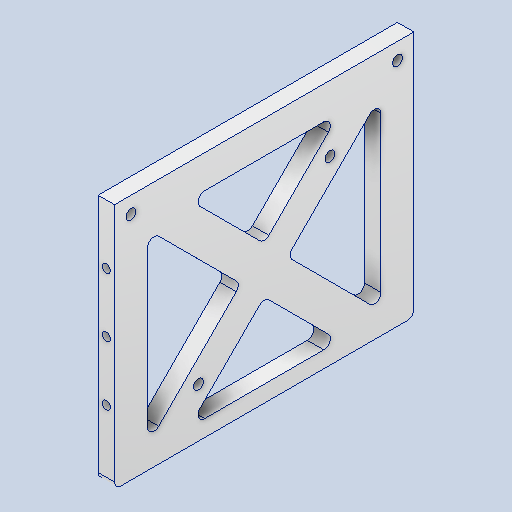
# Autodesk Inventor part: base_weel-v2-Plate-5
Saved by Autodesk Inventor 2025.2 (Build 292293000, 293)
## iProperties
Created: 2025-01-14
Part Number: base_weel-v2-Plate-5
Material: アルミニウム 6061
Document SubType Name: Modeling
Designer: haruy
Density: 2.7 g/cm^3
Appearance: アルミニウム - フラット
Author: haruy
Autodesk Inventor part; units mm, degrees
ref_plane "YZ Plane" through (0, 0, 0) normal (1, 0, 0) x (0, 1, 0)
ref_plane "XZ Plane" through (0, 0, 0) normal (0, 1, 0) x (-1, 0, 0)
ref_plane "XY Plane" through (0, 0, 0) normal (0, 0, 1) x (1, 0, 0)
derived "base_weel-v2-Sketch-Base.ipt"
sketch "スケッチ1" plane through (0, 0, 0) normal (1, 0, 0) x (0, 1, 0)
  line L0 (-315, 315) -> (315, 315)
  line L1 (315, 315) -> (315, -315)
  line L2 (315, -315) -> (-315, -315)
  line L3 (-315, -315) -> (-315, 315)
  line L4 (-315, 315) -> (315, -315) construction
  line L5 (315, 315) -> (-315, -315) construction
  line L6 (-295, 218) -> (-295, -202)
  line L7 (-295, -202) -> (-315, -202)
  line L8 (-315, -202) -> (-315, 210)
  line L9 (242, 315) -> (-242, 315)
  line L10 (-242, 315) -> (-242, 295)
  line L11 (-242, 295) -> (242, 295)
  line L12 (242, 295) -> (242, 315)
  line L13 (-295, 218) -> (-295, 315)
  line L14 (0, 0) -> (-956.5973, 0)
  circle A0 centre (0, 0) radius 400
  line L15 (-330, 25) -> (-380, 25)
  line L16 (-380, 25) -> (-380, -25)
  line L17 (-380, -25) -> (-330, -25)
  line L18 (-330, -25) -> (-330, 25)
  line L19 (0, 0) -> (0, -630.9179)
  line L20 (-315, 40) -> (-395, 40) construction
  line L21 (-395, 40) -> (-395, 30)
  line L22 (-395, 30) -> (-315, 30)
  line L23 (-315, 30) -> (-315, 40)
  line L24 (-395, 30) -> (-385, 30)
  line L25 (-385, 30) -> (-385, 0)
  line L26 (-385, 0) -> (-395, 0)
  line L27 (-395, 0) -> (-395, 30)
  line L28 (295, 202) -> (315, 202)
  line L29 (315, 202) -> (315, -202)
  line L30 (315, -202) -> (295, -202)
  line L31 (295, -202) -> (295, 202)
  line L32 (-222.2183, -315) -> (242, -315)
  line L33 (242, -315) -> (242, -295)
  line L34 (242, -295) -> (-242, -295)
  line L35 (315, 315) -> (0, 0)
  line L36 (315, 125) -> (315, 145)
  circle A1 centre (512, 0) radius 122.5
  circle A2 centre (179.6905, 0) radius 600
  circle A3 centre (541.6815, 0) radius 200
  circle A4 centre (0, 0) radius 10
  arc A5 (0, 150) -> (0, -150) centre (0, 0) ccw
  arc A6 (0, 140) -> (0, -140) centre (0, 0) ccw
  line L37 (-146.3272, 32.9904) -> (-136.572, 30.791)
  line L38 (-137.5812, 37.6817) -> (-140.4404, 25)
  line L39 (-140.4404, 25) -> (-145.318, 26.0997)
  line L40 (-145.318, 26.0997) -> (-142.4588, 38.7814)
  line L41 (-142.4588, 38.7814) -> (-137.5812, 37.6817)
  arc A7 (-29.1302, 142.0438) -> (-29.1302, -142.0438) centre (0, 0) ccw
  circle A8 centre (-151.4904, 39.2799) radius 6.5
  circle A9 centre (-129.0401, 34.2184) radius 6.5 construction
  circle A10 centre (-129.0401, 34.2184) radius 1.5 construction
  circle A11 centre (-151.4904, 39.2799) radius 1.5
  line L42 (-30.1668, 22.5) -> (-174.1362, 22.5)
  line L43 (-174.1362, 22.5) -> (-174.1362, 7.5)
  line L44 (-174.1362, 7.5) -> (-30.1668, 7.5)
  line L45 (-30.1668, 7.5) -> (-30.1668, 22.5)
  circle A12 centre (-129.0401, -34.2184) radius 6.5 construction
  circle A13 centre (-129.0401, -34.2184) radius 1.5 construction
  line L46 (-142.4588, -38.7814) -> (-137.5812, -37.6817)
  line L47 (-145.318, -26.0997) -> (-142.4588, -38.7814)
  line L48 (-137.5812, -37.6817) -> (-140.4404, -25)
  line L49 (-140.4404, -25) -> (-145.318, -26.0997)
  circle A14 centre (-151.4904, -39.2799) radius 6.5
  circle A15 centre (-151.4904, -39.2799) radius 1.5
  line L50 (-146.3272, -32.9904) -> (-136.572, -30.791)
  line L51 (-30.1668, -22.5) -> (-174.1362, -22.5)
  line L52 (-174.1362, -7.5) -> (-30.1668, -7.5)
  line L53 (-30.1668, -7.5) -> (-30.1668, -22.5)
  line L54 (-174.1362, -22.5) -> (-174.1362, -7.5)
  line L55 (-151.4904, 39.2799) -> (-129.0401, 34.2184) construction
  line L56 (-129.0401, 34.2184) -> (-129.59, 31.7796) construction
  line L57 (-129.59, 31.7796) -> (-152.0402, 36.8412) construction
  line L58 (-152.0402, 36.8412) -> (-151.4904, 39.2799) construction
  line L59 (-129.0401, 34.2184) -> (-151.4904, 39.2799) construction
  line L60 (-151.4904, 39.2799) -> (-150.9405, 41.7187) construction
  line L61 (-150.9405, 41.7187) -> (-128.4903, 36.6572) construction
  line L62 (-128.4903, 36.6572) -> (-129.0401, 34.2184) construction
  line L63 (-128.4903, 36.6572) -> (-129.59, 31.7796) construction
  line L64 (-129.59, 31.7796) -> (-117.8838, 29.1404) construction
  line L65 (-117.8838, 29.1404) -> (-116.7841, 34.0179) construction
  line L66 (-116.7841, 34.0179) -> (-128.4903, 36.6572) construction
  line L67 (-150.9405, 41.7187) -> (-152.0402, 36.8412) construction
  line L68 (-152.0402, 36.8412) -> (-163.7464, 39.4804) construction
  line L69 (-163.7464, 39.4804) -> (-162.6467, 44.358) construction
  line L70 (-162.6467, 44.358) -> (-150.9405, 41.7187) construction
  line L71 (-155.2683, 45.2572) -> (-128.9412, 39.3216)
  line L72 (-128.9412, 39.3216) -> (-132.2403, 24.6889)
  line L73 (-132.2403, 24.6889) -> (-158.5673, 30.6245)
  line L74 (-158.5673, 30.6245) -> (-155.2683, 45.2572)
  line L75 (-128.9412, -39.3216) -> (-132.2403, -24.6889)
  line L76 (-155.2683, -45.2572) -> (-128.9412, -39.3216)
  line L77 (-132.2403, -24.6889) -> (-158.5673, -30.6245)
  line L78 (-158.5673, -30.6245) -> (-155.2683, -45.2572)
  arc A16 (-132.2403, 24.6889) -> (-132.2403, -24.6889) centre (0, 0) ccw
  arc A17 (-158.5673, 30.6245) -> (-158.5673, -30.6245) centre (0, 0) ccw
  circle A18 centre (-152.5, 15) radius 1.25
  line L79 (-145, 0) -> (-145, 74.7382)
  circle A19 centre (-137.5, 15) radius 1.25
  circle A20 centre (-137.5, -15) radius 1.25
  circle A21 centre (-152.5, -15) radius 1.25
  line L80 (0, 0) -> (0, 140)
  line L81 (0, 0) -> (-47.8828, 131.557)
  line L82 (0, 140) -> (0, 150)
  line L83 (-137.5846, 25.8938) -> (-134.2855, 40.5265)
  line L84 (-137.5846, -25.8938) -> (-134.2855, -40.5265)
  circle A22 centre (0, 0) radius 20
  line L85 (295, 45) -> (-295, 45)
  line L86 (-295, 45) -> (-295, 25)
  line L87 (-295, 25) -> (295, 25)
  line L88 (295, 25) -> (295, 45)
  line L89 (-40, 295) -> (-50, 295)
  line L90 (-50, 295) -> (-50, 45)
  line L91 (-50, 45) -> (-40, 45)
  line L92 (-40, 45) -> (-40, 295)
  line L93 (-50, -295) -> (-50, -45)
  line L94 (-40, -45) -> (-40, -295)
  line L95 (295, -45) -> (-295, -45)
  line L96 (-295, -25) -> (295, -25)
  line L97 (-40, 45) -> (-40, -45)
  line L98 (40, 45) -> (40, -45)
  circle A23 centre (20, 35) radius 1.5
  circle A24 centre (-20, 35) radius 1.5
  circle A25 centre (-20, -35) radius 1.5
  circle A26 centre (20, -35) radius 1.5
  circle A27 centre (-45, 125) radius 1.5
  circle A28 centre (-45, 125) radius 5
  circle A29 centre (-130, 35) radius 5
  circle A30 centre (-130, 35) radius 1.5
  line L99 (-40, 134.1641) -> (-40, 125)
  line L100 (-50, 125) -> (-50, 130.767)
  line L101 (-137.7498, 25) -> (-127.5801, 30.6246)
  line L102 (-132.5707, 45) -> (-126.366, 38.4342)
  line L103 (-40, -134.1641) -> (-40, -125)
  circle A31 centre (-45, -125) radius 5
  circle A32 centre (-45, -125) radius 1.5
  line L104 (-50, -125) -> (-50, -130.767)
  line L105 (-132.5707, -45) -> (-126.366, -38.4342)
  circle A33 centre (-130, -35) radius 5
  circle A34 centre (-130, -35) radius 1.5
  line L106 (-137.7498, -25) -> (-127.5801, -30.6246)
  line L107 (-242, -295) -> (-242, -315)
  line L108 (242, 315) -> (222, 315)
  line L109 (222, 315) -> (222, 295)
  line L110 (222, 295) -> (242, 295)
  line L111 (242, 295) -> (242, 315)
  line L112 (242, -315) -> (222, -315)
  line L113 (222, -315) -> (222, -295)
  line L114 (222, -295) -> (242, -295)
  line L115 (242, -295) -> (242, -315)
  line L116 (197, 295) -> (295, 197)
  line L117 (295, 197) -> (284.3934, 186.3934)
  line L118 (284.3934, 186.3934) -> (186.3934, 284.3934)
  line L119 (186.3934, 284.3934) -> (197, 295)
  line L120 (197, 295) -> (197, 315)
  line L121 (197.9167, 294.0833) -> (187.3101, 283.4767)
  line L122 (198.2703, 272.5165) -> (272.5165, 198.2703)
  line L123 (272.5165, 198.2703) -> (231.5043, 157.2581)
  line L124 (231.5043, 157.2581) -> (157.2581, 231.5043)
  line L125 (157.2581, 231.5043) -> (198.2703, 272.5165)
  line L126 (290.9013, 201.0987) -> (280.2947, 190.4921)
  line L127 (93.7624, 295) -> (295, 93.7624)
  line L128 (295, 93.7624) -> (284.3934, 83.1558)
  line L129 (284.3934, 83.1558) -> (83.1558, 284.3934)
  line L130 (214.1802, 277.8198) -> (203.5736, 267.2132)
  line L131 (277.8198, 214.1802) -> (267.2132, 203.5736)
  circle A35 centre (199.6845, 281.7089) radius 1.5
  circle A36 centre (213.8266, 267.5668) radius 1.5
  line L132 (186.3934, 284.3934) -> (175.7868, 295)
  circle A37 centre (187, 305) radius 1.5
  circle A38 centre (177, 305) radius 1.5
  line L133 (172, 315) -> (172, 295)
  line L134 (93.7624, 295) -> (93.7624, 295)
  line L135 (93.7624, 295) -> (93.7624, 315)
  line L136 (83.1558, 284.3934) -> (72.5492, 295)
  line L137 (68.7624, 315) -> (68.7624, 295)
  line L138 (284.3934, 186.3934) -> (295, 175.7868)
  line L139 (295, 197) -> (315, 197)
  line L140 (295, 93.7624) -> (295, 93.7624)
  line L141 (284.3934, 83.1558) -> (295, 72.5492)
  line L142 (-197, 295) -> (-197, 315)
  line L143 (-172, 315) -> (-172, 295)
  line L144 (-93.7624, 295) -> (-93.7624, 315)
  line L145 (-68.7624, 315) -> (-68.7624, 295)
  line L146 (-83.1558, 284.3934) -> (-72.5492, 295)
  line L147 (-93.7624, 295) -> (-295, 93.7624)
  line L148 (-83.1558, 284.3934) -> (-93.7624, 295)
  line L149 (-284.3934, 83.1558) -> (-83.1558, 284.3934)
  line L150 (-295, 93.7624) -> (-284.3934, 83.1558)
  line L151 (-284.3934, 83.1558) -> (-295, 72.5492)
  line L152 (-272.5165, 198.2703) -> (-231.5043, 157.2581)
  line L153 (-157.2581, 231.5043) -> (-198.2703, 272.5165)
  line L154 (-284.3934, 186.3934) -> (-186.3934, 284.3934)
  line L155 (-186.3934, 284.3934) -> (-175.7868, 295)
  line L156 (-197, 295) -> (-295, 197)
  line L157 (-197.9167, 294.0833) -> (-187.3101, 283.4767)
  line L158 (-214.1802, 277.8198) -> (-203.5736, 267.2132)
  line L159 (-290.9013, 201.0987) -> (-280.2947, 190.4921)
  line L160 (-284.3934, 186.3934) -> (-295, 175.7868)
  line L161 (-295, 197) -> (-315, 197)
  line L162 (-93.7624, -295) -> (-295, -93.7624)
  line L163 (-284.3934, -83.1558) -> (-83.1558, -284.3934)
  line L164 (-295, -93.7624) -> (-284.3934, -83.1558)
  line L165 (-197, -295) -> (-295, -197)
  line L166 (-284.3934, -186.3934) -> (-186.3934, -284.3934)
  line L167 (-290.9013, -201.0987) -> (-280.2947, -190.4921)
  line L168 (-214.1802, -277.8198) -> (-203.5736, -267.2132)
  line L169 (-197.9167, -294.0833) -> (-187.3101, -283.4767)
  line L170 (-83.1558, -284.3934) -> (-93.7624, -295)
  line L171 (284.3934, -83.1558) -> (83.1558, -284.3934)
  line L172 (83.1558, -284.3934) -> (93.7624, -295)
  line L173 (93.7624, -295) -> (295, -93.7624)
  line L174 (284.3934, -186.3934) -> (186.3934, -284.3934)
  line L175 (197.9167, -294.0833) -> (187.3101, -283.4767)
  line L176 (197, -295) -> (295, -197)
  line L177 (290.9013, -201.0987) -> (280.2947, -190.4921)
  line L178 (295, -93.7624) -> (284.3934, -83.1558)
  line L179 (242, 295) -> (222, 295)
  arc A39 (0, 86) -> (0, -86) centre (0, 0) ccw construction
  circle A40 centre (-90.8667, 48.5) radius 21
  circle A41 centre (0, 0) radius 124
  circle A42 centre (-90.8667, 48.5) radius 17
  arc A43 (40.4951, 75.8693) -> (0, 86) centre (0, 0) ccw construction
  line L180 (-40, 45) -> (-50, 45)
  line L181 (-50, 45) -> (-50, -45)
  line L182 (-50, -45) -> (-40, -45)
  line L183 (-40, -45) -> (-40, 45)
  line L184 (-40, 295) -> (-50, 295)
  line L185 (-50, 295) -> (-50, 315)
  line L186 (-50, 315) -> (-40, 315)
  line L187 (-40, 315) -> (-40, 295)
  line L188 (-40, -295) -> (-50, -295)
  line L189 (-50, -295) -> (-50, -315)
  line L190 (-50, -315) -> (-40, -315)
  line L191 (-40, -315) -> (-40, -295)
  line L192 (40, -315) -> (40, -295)
  line L193 (50, -295) -> (50, -315)
  line L194 (50, -295) -> (50, -45)
  line L195 (40, -45) -> (40, -295)
  line L196 (40, -45) -> (40, 45)
  line L197 (50, 45) -> (50, -45)
  line L198 (40, 45) -> (40, 295)
  line L199 (50, 295) -> (50, 45)
  line L200 (40, 315) -> (40, 295)
  line L201 (50, 295) -> (50, 315)
  line L202 (-40.4092, 123.019) -> (-35, 135.5544)
  line L203 (-48.7417, 121.6834) -> (-55, 128.7439)
  line L204 (-40.4092, -123.019) -> (-35, -135.5544)
  line L205 (-48.7417, -121.6834) -> (-55, -128.7439)
  arc A44 (40.4951, 75.8693) -> (-40.4951, -75.8693) centre (0, 0) ccw
  circle A45 centre (0, 0) radius 86 construction
  circle A46 centre (0, 0) radius 78.5
  circle A47 centre (-45, 58) radius 1.5
  circle A48 centre (-45, 58) radius 5
  circle A49 centre (45, 58) radius 5
  circle A50 centre (45, 58) radius 1.5
  line L206 (46.5549, 53.2479) -> (55, 56.0112)
  line L207 (40.325, 56.2267) -> (35, 70.2656)
  line L208 (50, 60.5165) -> (50, 69.9714)
  arc A51 (50, 69.9714) -> (40.4951, 75.8693) centre (0, 0) ccw
  line L209 (-40.325, 56.2267) -> (-35, 70.2656)
  line L210 (-46.5549, 53.2479) -> (-55, 56.0112)
  line L211 (-40.325, -56.2267) -> (-35, -70.2656) construction
  circle A52 centre (-45, -58) radius 5
  line L212 (-46.5549, -53.2479) -> (-55, -56.0112)
  circle A53 centre (-45, -58) radius 1.5
  line L213 (-40, -67.5444) -> (-40, -76.1315)
  arc A54 (-40.526, -75.8528) -> (-40, -76.1315) centre (0, 0) ccw
  line L214 (-40, -76.1315) -> (-40, -58)
  line L215 (222.6655, 269.3345) -> (212.0589, 258.7279)
  line L216 (269.3345, 222.6655) -> (258.7279, 212.0589)
  circle A55 centre (267.5668, 213.8266) radius 1.5
  circle A56 centre (281.7089, 199.6845) radius 1.5
  line L217 (294.0833, 197.9167) -> (283.4767, 187.3101)
  line L218 (315, 172) -> (295, 172)
  circle A57 centre (305, 177) radius 1.5
  circle A58 centre (305, 187) radius 1.5
  line L219 (295, 197) -> (315, 197)
  circle A59 centre (83.7624, 305) radius 1.5
  circle A60 centre (73.7624, 305) radius 1.5
  line L220 (197.9167, 294.0833) -> (94.6791, 294.0833)
  line L221 (187.3101, 283.4767) -> (84.0725, 283.4767)
  line L222 (94.6791, 294.0833) -> (84.0725, 283.4767)
  circle A61 centre (96.4469, 281.7089) radius 1.5
  circle A62 centre (110.5891, 267.5668) radius 1.5
  line L223 (119.4279, 269.3345) -> (108.8213, 258.7279)
  line L224 (295, 93.7624) -> (315, 93.7624)
  line L225 (315, 68.7624) -> (295, 68.7624)
  circle A63 centre (305, 73.7624) radius 1.5
  circle A64 centre (305, 83.7624) radius 1.5
  line L226 (294.0833, 94.6791) -> (283.4767, 84.0725)
  circle A65 centre (281.7089, 96.4469) radius 1.5
  circle A66 centre (267.5668, 110.5891) radius 1.5
  line L227 (269.3345, 119.4279) -> (258.7279, 108.8213)
  line L228 (-197, 295) -> (-197, 315)
  line L229 (-172, 315) -> (-172, 295)
  circle A67 centre (-177, 305) radius 1.5
  circle A68 centre (-187, 305) radius 1.5
  line L230 (-197.9167, 294.0833) -> (-187.3101, 283.4767)
  circle A69 centre (-199.6845, 281.7089) radius 1.5
  line L231 (-214.1802, 277.8198) -> (-203.5736, 267.2132)
  circle A70 centre (-213.8266, 267.5668) radius 1.5
  line L232 (-222.6655, 269.3345) -> (-212.0589, 258.7279)
  circle A71 centre (-267.5668, 213.8266) radius 1.5
  line L233 (-269.3345, 222.6655) -> (-258.7279, 212.0589)
  circle A72 centre (-281.7089, 199.6845) radius 1.5
  line L234 (-294.0833, 197.9167) -> (-283.4767, 187.3101)
  line L235 (-295, 197) -> (-315, 197)
  circle A73 centre (-305, 187) radius 1.5
  circle A74 centre (-305, 177) radius 1.5
  line L236 (-315, 172) -> (-295, 172)
  line L237 (-295, 93.7624) -> (-315, 93.7624)
  line L238 (-315, 68.7624) -> (-295, 68.7624)
  circle A75 centre (-305, 73.7624) radius 1.5
  circle A76 centre (-305, 83.7624) radius 1.5
  line L239 (-294.0833, 94.6791) -> (-283.4767, 84.0725)
  circle A77 centre (-281.7089, 96.4469) radius 1.5
  circle A78 centre (-267.5668, 110.5891) radius 1.5
  line L240 (-269.3345, 119.4279) -> (-258.7279, 108.8213)
  line L241 (-119.4279, 269.3345) -> (-108.8213, 258.7279)
  circle A79 centre (-110.5891, 267.5668) radius 1.5
  circle A80 centre (-96.4469, 281.7089) radius 1.5
  line L242 (-94.6791, 294.0833) -> (-84.0725, 283.4767)
  line L243 (-93.7624, 295) -> (-93.7624, 315)
  line L244 (-68.7624, 315) -> (-68.7624, 295)
  circle A81 centre (-73.7624, 305) radius 1.5
  circle A82 centre (-83.7624, 305) radius 1.5
  line L245 (-295, -197) -> (-315, -197)
  circle A83 centre (-305, -187) radius 1.5
  circle A84 centre (-305, -177) radius 1.5
  line L246 (-315, -172) -> (-295, -172)
  line L247 (-294.0833, -197.9167) -> (-283.4767, -187.3101)
  circle A85 centre (-281.7089, -199.6845) radius 1.5
  circle A86 centre (-267.5668, -213.8266) radius 1.5
  line L248 (-269.3345, -222.6655) -> (-258.7279, -212.0589)
  line L249 (-222.6655, -269.3345) -> (-212.0589, -258.7279)
  circle A87 centre (-213.8266, -267.5668) radius 1.5
  circle A88 centre (-199.6845, -281.7089) radius 1.5
  line L250 (-197.9167, -294.0833) -> (-187.3101, -283.4767)
  line L251 (-197, -295) -> (-197, -315)
  circle A89 centre (-187, -305) radius 1.5
  circle A90 centre (-177, -305) radius 1.5
  line L252 (-172, -315) -> (-172, -295)
  line L253 (-295, -93.7624) -> (-315, -93.7624)
  circle A91 centre (-305, -83.7624) radius 1.5
  circle A92 centre (-305, -73.7624) radius 1.5
  line L254 (-315, -68.7624) -> (-295, -68.7624)
  line L255 (-294.0833, -94.6791) -> (-283.4767, -84.0725)
  circle A93 centre (-281.7089, -96.4469) radius 1.5
  circle A94 centre (-267.5668, -110.5891) radius 1.5
  line L256 (-269.3345, -119.4279) -> (-258.7279, -108.8213)
  line L257 (-119.4279, -269.3345) -> (-108.8213, -258.7279)
  circle A95 centre (-110.5891, -267.5668) radius 1.5
  circle A96 centre (-96.4469, -281.7089) radius 1.5
  line L258 (-94.6791, -294.0833) -> (-84.0725, -283.4767)
  line L259 (-93.7624, -295) -> (-93.7624, -315)
  circle A97 centre (-83.7624, -305) radius 1.5
  circle A98 centre (-73.7624, -305) radius 1.5
  line L260 (-68.7624, -315) -> (-68.7624, -295)
  line L261 (68.7624, -315) -> (68.7624, -295)
  circle A99 centre (73.7624, -305) radius 1.5
  circle A100 centre (83.7624, -305) radius 1.5
  line L262 (93.7624, -295) -> (93.7624, -315)
  line L263 (94.6791, -294.0833) -> (84.0725, -283.4767)
  circle A101 centre (96.4469, -281.7089) radius 1.5
  circle A102 centre (110.5891, -267.5668) radius 1.5
  line L264 (119.4279, -269.3345) -> (108.8213, -258.7279)
  line L265 (172, -315) -> (172, -295)
  circle A103 centre (177, -305) radius 1.5
  circle A104 centre (187, -305) radius 1.5
  line L266 (197, -295) -> (197, -315)
  line L267 (197.9167, -294.0833) -> (187.3101, -283.4767)
  circle A105 centre (199.6845, -281.7089) radius 1.5
  circle A106 centre (213.8266, -267.5668) radius 1.5
  line L268 (222.6655, -269.3345) -> (212.0589, -258.7279)
  line L269 (269.3345, -222.6655) -> (258.7279, -212.0589)
  circle A107 centre (267.5668, -213.8266) radius 1.5
  circle A108 centre (281.7089, -199.6845) radius 1.5
  line L270 (294.0833, -197.9167) -> (283.4767, -187.3101)
  line L271 (295, -197) -> (315, -197)
  circle A109 centre (305, -187) radius 1.5
  circle A110 centre (305, -177) radius 1.5
  line L272 (315, -172) -> (295, -172)
  line L273 (295, -93.7624) -> (315, -93.7624)
  circle A111 centre (305, -83.7624) radius 1.5
  circle A112 centre (305, -73.7624) radius 1.5
  line L274 (315, -68.7624) -> (295, -68.7624)
  line L275 (294.0833, -94.6791) -> (283.4767, -84.0725)
  circle A113 centre (281.7089, -96.4469) radius 1.5
  line L276 (269.3345, -119.4279) -> (258.7279, -108.8213)
  circle A114 centre (267.5668, -110.5891) radius 1.5
  line L277 (-295, 202) -> (-315, 202)
  line L278 (265, 45) -> (265, 25)
  circle A115 centre (275, 35) radius 1.5
  circle A116 centre (285, 35) radius 1.5
  circle A117 centre (305, 35) radius 1.5
  circle A118 centre (305, 25) radius 1.5
  line L279 (295, 25) -> (315, 25)
  line L280 (265, -45) -> (265, -25)
  circle A119 centre (275, -35) radius 1.5
  circle A120 centre (285, -35) radius 1.5
  circle A121 centre (305, -35) radius 1.5
  circle A122 centre (305, -25) radius 1.5
  circle A123 centre (-305, -25) radius 1.5
  circle A124 centre (-305, -35) radius 1.5
  circle A125 centre (-285, -35) radius 1.5
  circle A126 centre (-275, -35) radius 1.5
  line L281 (-265, -45) -> (-265, -25)
  line L282 (-265, 45) -> (-265, 25)
  circle A127 centre (-275, 35) radius 1.5
  circle A128 centre (-285, 35) radius 1.5
  circle A129 centre (-305, 35) radius 1.5
  circle A130 centre (-305, 25) radius 1.5
  circle A131 centre (48, 345) radius 44
  circle A132 centre (-50, 345) radius 44
  circle A133 centre (-50, 345) radius 15
  line L283 (295, 45) -> (315, 45)
  line L284 (295, 15) -> (315, 15)
  line L285 (-315, 45.5) -> (-390, 45.5)
  line L286 (-390, 45.5) -> (-390, 0)
  line L287 (-390, 0) -> (-315, 0)
  line L288 (-315, 0) -> (-315, 45.5)
  circle A134 centre (-305, 48) radius 1.5
  line L289 (-315, -45.5) -> (-390, -45.5)
  line L290 (-390, -45.5) -> (-390, 0)
  circle A135 centre (-375, 20) radius 1.5
  circle A136 centre (-335, -20) radius 1.5
  line L291 (-330, 25) -> (-380, -25)
  line L292 (-380, 25) -> (-330, -25)
  line L293 (-385, 30) -> (-385, 45.5)
  line L294 (-315, 35.5) -> (-385, 35.5)
  line L295 (-385, -30) -> (-385, 0)
  line L296 (-385, -30) -> (-385, -45.5)
  line L297 (-315, -35.5) -> (-385, -35.5)
  line L298 (-380, 25) -> (-385, 30)
  line L299 (-330, 25) -> (-325, 30)
  line L300 (-380, -25) -> (-385, -30)
  line L301 (-330, -25) -> (-325, -30)
  line L302 (-328.0327, -34.0384) -> (-333.5355, -28.5355)
  line L303 (-333.5355, -28.5355) -> (-383.5355, 21.4645)
  line L304 (-383.5355, 21.4645) -> (-390, 27.9289)
  line L305 (-390, 27.9289) -> (-390, 45.5)
  line L306 (-388.5355, -26.4645) -> (-383.5355, -21.4645)
  line L307 (-383.5355, -21.4645) -> (-333.5355, 28.5355)
  line L308 (-333.5355, 28.5355) -> (-328.5356, 33.5354)
  line L309 (-390, -40.5) -> (-300.5339, -40.5) construction
  line L310 (-321.9673, -25.9616) -> (-326.4645, -21.4645)
  line L311 (-326.4645, -21.4645) -> (-376.4645, 28.5355)
  line L312 (-376.4645, 28.5355) -> (-380, 32.0711)
  line L313 (-380, 32.0711) -> (-380, 45.5)
  line L314 (-381.4645, -33.5355) -> (-376.4645, -28.5355)
  line L315 (-376.4645, -28.5355) -> (-326.4645, 21.4645)
  line L316 (-326.4645, 21.4645) -> (-321.4645, 26.4645)
  line L317 (-325, 45.5) -> (-325, -40.5)
  line L318 (-321.4645, 26.4645) -> (-325, 22.9289)
  line L319 (-328.5356, 33.5354) -> (-326.5711, 35.5)
  line L320 (-380, 32.0711) -> (-383.4289, 35.5)
  line L321 (-381.4645, -33.5355) -> (-383.4289, -35.5)
  line L322 (-321.9673, -25.9616) -> (-325, -22.9289)
  line L323 (-328.0327, -34.0384) -> (-326.5711, -35.5)
  circle A137 centre (-320, 40.5) radius 5
  circle A138 centre (-320, 40.5) radius 1.5
  circle A139 centre (-320, -40.5) radius 1.5
  circle A140 centre (-305, -48) radius 1.5
  line L324 (114.7878, 210) -> (54.7878, 210)
  line L325 (54.7878, 210) -> (54.7878, 270)
  line L326 (54.7878, 270) -> (114.7878, 270)
  line L327 (114.7878, 270) -> (114.7878, 210)
  line L328 (34.7878, 210) -> (-25.2122, 210)
  line L329 (-25.2122, 210) -> (-25.2122, 270)
  line L330 (-25.2122, 270) -> (34.7878, 270)
  line L331 (34.7878, 270) -> (34.7878, 210)
  line L332 (-45.2122, 250) -> (-115.2122, 250)
  line L333 (-115.2122, 250) -> (-115.2122, 266)
  line L334 (-115.2122, 266) -> (-45.2122, 266)
  line L335 (-45.2122, 266) -> (-45.2122, 250)
  line L336 (-50.2122, 214) -> (-110.2122, 214)
  line L337 (-110.2122, 214) -> (-110.2122, 230)
  line L338 (-110.2122, 230) -> (-50.2122, 230)
  line L339 (-50.2122, 230) -> (-50.2122, 214)
  circle A141 centre (0, 0) radius 175.5
  line L340 (-185, -89) -> (-302, -89)
  line L341 (-302, -89) -> (-302, 89)
  line L342 (-302, 89) -> (-185, 89)
  line L343 (-185, 89) -> (-185, -89)
  line L344 (287, -17.7878) -> (205, -17.7878)
  line L345 (205, -17.7878) -> (205, 79.2122)
  line L346 (205, 79.2122) -> (287, 79.2122)
  line L347 (287, 79.2122) -> (287, -17.7878)
  line L348 (284.5, -114.7878) -> (207.5, -114.7878)
  line L349 (207.5, -114.7878) -> (207.5, -37.7878)
  line L350 (207.5, -37.7878) -> (284.5, -37.7878)
  line L351 (284.5, -37.7878) -> (284.5, -114.7878)
  line L352 (281, 99.2122) -> (211, 99.2122)
  line L353 (211, 99.2122) -> (211, 115.2122)
  line L354 (211, 115.2122) -> (281, 115.2122)
  line L355 (281, 115.2122) -> (281, 99.2122)
  line L356 (137.7122, 315) -> (-137.7122, 315)
  line L357 (-137.7122, 315) -> (-137.7122, 185)
  line L358 (-137.7122, 185) -> (137.7122, 185)
  line L359 (137.7122, 185) -> (137.7122, 315)
  line L360 (315, -137.7122) -> (185, -137.7122)
  line L361 (185, -137.7122) -> (185, 137.7122)
  line L362 (185, 137.7122) -> (315, 137.7122)
  line L363 (315, 137.7122) -> (315, -137.7122)
  line L364 (258.7782, 137.7122) -> (278.7782, 137.7122)
  line L365 (278.7782, 137.7122) -> (278.7782, 127.7122)
  line L366 (278.7782, 127.7122) -> (258.7782, 127.7122)
  line L367 (258.7782, 127.7122) -> (258.7782, 137.7122)
  circle A142 centre (268.7782, 132.7122) radius 1.5
  line L368 (278.7782, 137.7122) -> (231.1981, 137.7122)
  line L369 (231.1981, 137.7122) -> (231.1981, 147.7122)
  line L370 (231.1981, 147.7122) -> (278.7782, 147.7122)
  line L371 (278.7782, 147.7122) -> (278.7782, 137.7122)
  line L372 (255.1924, 112.3568) -> (233.9792, 133.57)
  line L373 (233.9792, 133.57) -> (230.4437, 130.0345)
  line L374 (230.4437, 130.0345) -> (251.6569, 108.8213)
  line L375 (251.6569, 108.8213) -> (255.1924, 112.3568)
  line L376 (288.78, 89.3758) -> (114.1246, 264.0312)
  line L377 (269.3345, 126.499) -> (265.799, 122.9634)
  line L378 (248.1213, 147.7122) -> (269.3345, 126.499)
  line L379 (244.5858, 144.1766) -> (248.1213, 147.7122)
  circle A143 centre (268.7782, 132.7122) radius 4
  line L380 (233.9792, 133.57) -> (244.5858, 144.1766)
  line L381 (-330, 143.5) -> (-340, 143.5)
  line L382 (-340, 143.5) -> (-340, -143.5)
  line L383 (-340, -143.5) -> (-330, -143.5)
  line L384 (-330, -143.5) -> (-330, 143.5)
  line L385 (-315, 119) -> (-295, 119)
  line L386 (-295, 119) -> (-295, 104)
  line L387 (-295, 104) -> (-315, 104)
  line L388 (-315, 104) -> (-315, 119)
  line L389 (-315, 153.5) -> (-325, 153.5)
  line L390 (-325, 153.5) -> (-325, 0)
  line L391 (-325, 0) -> (-315, 0)
  line L392 (-315, 0) -> (-315, 153.5)
  line L393 (-340, 133.5) -> (-345, 133.5)
  line L394 (-345, 133.5) -> (-345, 143.5)
  line L395 (-345, 143.5) -> (-340, 143.5)
  line L396 (-340, 143.5) -> (-340, 133.5)
  line L397 (-330, 133.5) -> (-325, 133.5)
  line L398 (-325, 133.5) -> (-325, 143.5)
  line L399 (-325, 143.5) -> (-330, 143.5)
  line L400 (-330, 143.5) -> (-330, 133.5)
  line L401 (-325, 153.5) -> (-345, 153.5)
  line L402 (-345, 153.5) -> (-345, 143.5)
  line L403 (-345, 143.5) -> (-325, 143.5)
  line L404 (-325, 143.5) -> (-325, 153.5)
  line L405 (-295, 104) -> (-345, 104)
  line L406 (-345, 104) -> (-345, 98)
  line L407 (-345, 98) -> (-295, 98)
  line L408 (-295, 98) -> (-295, 104)
  line L409 (185, -25) -> (180, -25)
  line L410 (180, -25) -> (180, -15)
  line L411 (180, -15) -> (185, -15)
  line L412 (185, -15) -> (185, -25)
  line L413 (185, -25) -> (195, -25)
  line L414 (195, -25) -> (195, -15)
  line L415 (195, -15) -> (185, -15)
  line L416 (185, -15) -> (185, -25)
  line L417 (40, 180) -> (30, 180)
  line L418 (30, 180) -> (30, 195)
  line L419 (30, 195) -> (40, 195)
  line L420 (40, 195) -> (40, 180)
  circle A144 centre (-132.7122, 268.7782) radius 1.5
  circle A145 centre (132.7122, 268.7782) radius 1.5
  line L421 (-243.5, 89) -> (-243.5, -89)
  circle A146 centre (-214, 35) radius 1.5
  circle A147 centre (-214, -35) radius 1.5
  line L422 (-214, 89) -> (-214, -89)
  line L423 (-246, 89) -> (-246, -89)
  circle A148 centre (-254.5, 35) radius 4
  circle A149 centre (-254.5, -35) radius 4
  circle A150 centre (0, 0) radius 100
  circle A151 centre (-134.1671, -14.9726) radius 5
  circle A152 centre (-134.1671, -14.9726) radius 1.25
  circle A153 centre (-134.9074, -5) radius 5
  circle A154 centre (-134.9074, -5) radius 1.25
  point P0 (-141.4496, 31.8907)
  point P1 (-129.0401, 34.2184)
  point P2 (-150, 0)
  point P3 (-242, 305)
  point P4 (-295, 93.7624)
  point P5 (-161.4975, 0)
  point P6 (305, 25)
  point P7 (295, 35)
  point P8 (-385, 22.9289)
  point P9 (-362.0711, 0)
  point P10 (-385, -22.9289)
  point P11 (-355, 7.0711)
  point P12 (-347.9289, 0)
  point P13 (-325, 22.9289)
  point P14 (-355, -7.0711)
  dimension "d1" = 3
  dimension "d2" = 5
  dimension "d3" = 5
  dimension "d4" = 3
  dimension "d5" = 5
  dimension "d6" = 5
  dimension "d7" = 10
  dimension "d8" = 5
  dimension "d9" = 5
  dimension "d10" = 5
  dimension "d11" = 5
  dimension "d12" = 10
  dimension "d16" = 10
  dimension "d17" = 3
  measures "d1" diameter of A135
  measures "d2" distance from line of A135.centre L16
  measures "d3" distance from line of A135.centre L15
  measures "d4" diameter of A136
  measures "d5" distance from line of A136.centre L18
  measures "d6" distance from line of L17 A136.centre
  measures "d7" distance between parallel lines of L285 L294
  measures "d8" distance between parallel lines of L292 L303
  measures "d9" distance between parallel lines of L291 L307
  measures "d10" distance between parallel lines of L292 L311
  measures "d11" distance between parallel lines of L291 L315
  measures "d12" distance between parallel lines of L317 L8
  measures "d16" diameter of A137
  measures "d17" diameter of A138
extrude "押し出し1" add sketch "スケッチ1" against normal blind 5 contours L286 L304 L25 L14 | L14 L295 L296 L289 L290 | L286 L22 L25 L304 | L286 L285 L293 L22 | L25 L298 L16 L303 L304 | L306 L307 L16 L300 L295 | L296 L297 L382 L289 | L293 L294 L320 L312 L22 | L22 L312 L311 L15 L298 | L307 L292 L14 | L14 L291 L303 | L303 L291 L16 L307 | L303 L16 L292 A135 L307 | L300 L17 L315 L314 L321 L297 L296 | L382 L297 L384 L289 | L293 L285 L313 L294 | L15 L311 L307 L292 A135 | L291 L311 L14 | L292 L307 L311 L291 | L292 L315 L303 L291 | L14 L315 L292 | L303 L315 L17 L291 | L384 L297 L3 L289 | L285 L382 L294 L313 | L311 L382 L292 L315 | L311 L291 L382 L315 | L311 L307 L382 L291 | L292 L382 L303 L315 | L308 L384 L22 | L22 L384 L15 L307 L308 | L382 L285 L384 L294 | L311 L18 L292 A136 L382 | L382 L291 L18 L315 | L382 L307 L15 L291 | L292 A136 L17 L303 L382 | L297 L317 L14 L3 | L323 L302 L384 L301 L317 L297 | L302 L303 L17 L384 | L384 L308 L319 L294 L317 L22 | L22 L299 L384 | L384 L285 L317 L294 | L285 A137 L317 | L311 L310 L317 L301 L18 | L18 L299 L317 L316 L315 | L14 L317 L22 L3 | L317 L294 L3 L22 | L3 A137 L285 | A137 | A137 L294 L317 | L3 L294 A137 | A138 | A139
fillet "フィレット1" radius 2 12 edges at (-2.5, -383.4289, 35.5) (-2.5, -355, 7.0711) (-2.5, -326.5711, 35.5) (-2.5, -385, 22.9289) (-2.5, -362.0711, 0) (-2.5, -385, -22.9289) (-2.5, -383.4289, -35.5) (-2.5, -355, -7.0711) (-2.5, -326.5711, -35.5) (-2.5, -325, -22.9289) (-2.5, -347.9289, 0) (-2.5, -325, 22.9289)
extrude "押し出し2" cut sketch "スケッチ1" against normal blind 5 contours A138 | A139
sketch "スケッチ2" plane through (0, -390, 45.5) normal (0, 0, 1) x (1, 0, 0)
  line L0 (0, 75) -> (-5, 75) projected
  line L1 (-5, 0) -> (-5, 75) projected
  point P0 (0, 390)
  point P1 (-2.5, 57)
  point P2 (-2.5, 39)
  point P3 (-2.5, 21)
  dimension "d20" = 18
  dimension "d21" = 18
  dimension "d22" = 18
  dimension "d23" = 2.5
  dimension "d24" = 2.5
  dimension "d25" = 2.5
  measures "d20" distance from line of point (-2.5, 57) L0
  measures "d21" distance of point (-2.5, 39) point (-2.5, 57)
  measures "d22" distance of point (-2.5, 21) point (-2.5, 39)
  measures "d23" distance from line of point (-2.5, 57) L1
  measures "d24" distance from line of point (-2.5, 39) L1
  measures "d25" distance from line of point (-2.5, 21) L1
hole "穴1" at (-2.5, -333, 45.5) at (-2.5, -351, 45.5) at (-2.5, -369, 45.5) direction (0, 0, -1) diameter 2.5 depth 5 tip angle 118
thread "ねじ1" size "M2.5x0.45" class "6H" standard "ANSI Metric M Profile" full length
thread "ねじ2" size "M2.5x0.45" class "6H" standard "ANSI Metric M Profile" full length
thread "ねじ3" size "M2.5x0.45" class "6H" standard "ANSI Metric M Profile" full length
ref_plane "作業平面1" through (0, -390, 0) normal (0, 0, 1) x (1, 0, 0)
mirror "ミラー1" about plane through (0, -390, 0) normal (0, 0, 1) of "穴1"
fillet "フィレット2" radius 2 2 edges at (-2.5, -390, 45.5) (-2.5, -390, -45.5)
equation "\"d3\" = d2"
equation "\"d6\" = d5"
equation "\"d21\" = d20"
equation "\"d22\" = d20"
equation "\"d24\" = d23"
equation "\"d25\" = d23"
